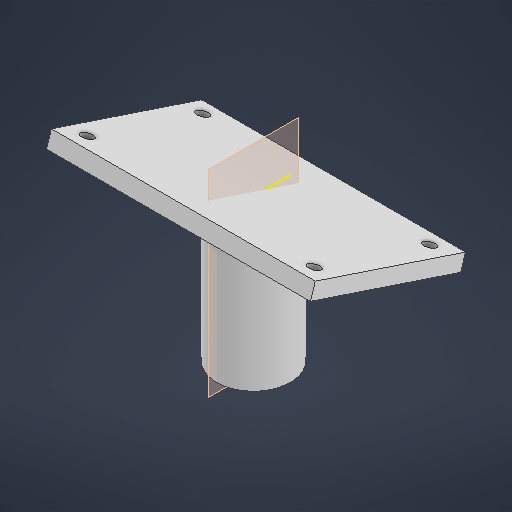
# Autodesk Inventor part: подставка для драйвер хаба
Saved by Autodesk Inventor 2026.2 (Build 302298000, 298)
## iProperties
Created: 2026-01-06
Part Number: подставка для драйвер хаба
Material: Типовые
Document SubType Name: Modeling
Designer: Phantom
Density: 1 g/cm^3
Appearance: По умолчанию
Author: Phantom
Autodesk Inventor part; units mm, degrees
ref_plane "YZ Plane" through (0, 0, 0) normal (1, 0, 0) x (0, 1, 0)
ref_plane "XZ Plane" through (0, 0, 0) normal (0, 1, 0) x (-1, 0, 0)
ref_plane "XY Plane" through (0, 0, 0) normal (0, 0, 1) x (1, 0, 0)
sketch "Эскиз1" plane through (0, 0, 0) normal (0, 1, 0) x (-1, 0, 0)
  circle A0 centre (0, 0) radius 11.5
  circle A1 centre (0, 0) radius 14
  dimension "d0" = 23
  dimension "d1" = 28
  constraints: 2 centre point, 2 coincident
  measures "d0" diameter of A0
  measures "d1" diameter of A1
extrude "Выдавливание1" add sketch "Эскиз1" along normal blind 40
sketch "Эскиз6" plane through (0, 40, 0) normal (0, 1, 0) x (1, 0, 0)
  circle A0 centre (0, 0) radius 14
  circle A1 centre (0, 0) radius 11.5 projected
  circle A2 centre (0, 0) radius 12
  circle A3 centre (0, 0) radius 12
  constraints: 3 centre point, 3 coincident, 1 concentric
extrude "Выдавливание5" add sketch "Эскиз6" along normal blind 14 contours A0 | A2
ref_plane "РабПлоскость1" through (0, 54, 11.8651) normal (1, 0, 0) x (0, 0, -1)
sketch "Эскиз8" plane through (0, 54, 11.8651) normal (1, 0, 0) x (0, 0, -1)
  line L0 (25.8651, 0) -> (-2.1349, 0) projected
  point P0 (11.8651, -54)
sketch "Эскиз9" plane through (0, 54, 11.8651) normal (1, 0, 0) x (0, 0, -1)
  line L0 (25.8651, 0) -> (-2.1349, 0) projected
  line L1 (-2.1349, 0) -> (27.9474, -10)
  line L2 (27.9474, -10) -> (27.9474, 0)
  line L3 (25.8651, -54) -> (25.8651, 0) projected
  line L4 (27.9474, 0) -> (-2.1349, 0)
  line L5 (0.3651, 0) -> (23.3651, 0) projected
  point P0 (11.8651, -54)
  dimension "d30" = 10
  constraints: 6 end point, 1 collinear, 1 parallel
  measures "d30" distance of L1.end L2.end
extrude "Выдавливание7" cut sketch "Эскиз9" along normal mid plane 70
sketch "Эскиз10" plane through (0, 49.3461, 0) normal (0, 0.9489425, -0.3154492) x (1, 0, 0)
  line L0 (50, -30) -> (-50, -30)
  line L1 (-50, -30) -> (-50, 30)
  line L2 (-50, 30) -> (50, 30)
  line L3 (50, 30) -> (50, -30)
  line L4 (50, -30) -> (-50, 30) construction
  line L5 (-50, -30) -> (50, 30) construction
  point P0 (0, 15.5662)
  point P1 (0, 0)
  dimension "d33" = 100
  dimension "d34" = 60
  constraints: 12 end point, 2 midpoint, 2 parallel, 1 horizontal, 1 perpendicular
  measures "d33" distance of L1.end L2.end
  measures "d34" distance of L0.end L1.end
extrude "Выдавливание8" add sketch "Эскиз10" along normal blind 6
sketch "Эскиз11" plane through (0, 55.0397, -1.8927) normal (0, 0.9489425, -0.3154492) x (1, 0, 0)
  circle A0 centre (-43, -23) radius 2.25
  line L0 (-50, 30) -> (-50, -30) projected
  line L1 (-50, -30) -> (50, -30) projected
  circle A1 centre (-43, 23) radius 2.25
  line L2 (50, 30) -> (-50, 30) projected
  circle A2 centre (43, -23) radius 2.25
  line L3 (50, -30) -> (50, 30) projected
  circle A3 centre (43, 23) radius 2.25
  point P0 (0, 15.5662)
  dimension "d37" = 4.5
  dimension "d38" = 7
  dimension "d39" = 7
  dimension "d40" = 4.5
  dimension "d41" = 7
  dimension "d42" = 7
  dimension "d43" = 4.5
  dimension "d44" = 7
  dimension "d45" = 7
  dimension "d46" = 4.5
  dimension "d47" = 7
  dimension "d48" = 7
  constraints: 4 centre point
  measures "d37" diameter of A0
  measures "d38" distance from line of L0 A0.centre
  measures "d39" distance from line of L1 A0.centre
  measures "d40" diameter of A1
  measures "d41" distance from line of L0 A1.centre
  measures "d42" distance from line of L2 A1.centre
  measures "d43" diameter of A2
  measures "d44" distance from line of L1 A2.centre
  measures "d45" distance from line of L3 A2.centre
  measures "d46" diameter of A3
  measures "d47" distance from line of L2 A3.centre
  measures "d48" distance from line of L3 A3.centre
extrude "Выдавливание9" cut sketch "Эскиз11" against normal blind 6 contours A0 | A1 | A2 | A3
